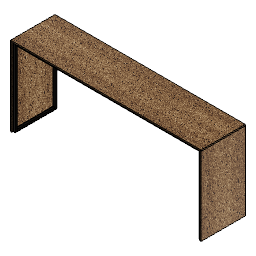
table de lit (Autodesk Fusion 360 design; units mm, degrees)
Autodesk Fusion 360 part; units mm, degrees
sketch "Sketch1" plane through (0, 0, 0) normal (0, 0, 1) x (1, 0, 0) in component "Plateau"
  line L0 (0, 0) -> (1800, 0)
  line L1 (1800, 0) -> (1800, 420)
  line L2 (1800, 420) -> (0, 420)
  line L3 (0, 420) -> (0, 0)
  dimension "d8" = 1800
  dimension "d9" = 420
  constraint horizontal L0
  constraint vertical L1
  constraint horizontal L2
  constraint vertical L3
  constraint coincident L0.start L3.end
  measures "d8" distance of L0.start L0.end
  measures "d9" distance of L0.start L2.end
extrude "Extrude1" add sketch "Sketch1" along normal blind 12 makes body 1 in component "Plateau"
sketch "Sketch1 (2)" plane through (0, 0, 0) normal (0, 0, 1) x (1, 0, 0) in component "Pied"
  line L0 (0, 0) -> (20, 0)
  line L1 (20, 0) -> (20, 20)
  line L2 (20, 20) -> (0, 20)
  line L3 (0, 20) -> (0, 0)
  dimension "d12" = 20
  dimension "d13" = 20
  constraint horizontal L0
  constraint vertical L1
  constraint horizontal L2
  constraint vertical L3
  constraint coincident L0.start L3.end
  measures "d12" distance of L0.start L0.end
  measures "d13" distance of L0.start L2.end
extrude "Extrude1'" add sketch "Sketch1 (2)" along normal blind 738 separate body makes body 2 in component "Pied"
shell "Shell1" thickness 2 removed faces 2 at (6.6667, 13.3333, 738) at (6.6667, 13.3333, 0) on bodies 2 in component "Pied"
pattern_linear "R-Pattern1" count 2 spacing 1756 along (1, 0, 0) count 2 spacing 376 along (0, 1, 0) of bodies 2 makes body 3 at (1756, 13.3333, 246) makes body 4 at (0, 389.3333, 246) makes body 5 at (1756, 389.3333, 246) in component "Pied"
sketch "Sketch2" plane through (0, 0, 738) normal (0, 0, 1) x (-1, 0, 0) in component "Pied"
  line L0 (-2, -18) -> (-18, -18)
  line L1 (-18, -18) -> (-18, -2)
  line L2 (-18, -2) -> (-2, -2)
  line L3 (-2, -2) -> (-2, -18)
  line L4 (0, -20) -> (0, 0)
  line L5 (0, 0) -> (-20, 0)
  line L6 (-20, 0) -> (-20, -20)
  line L7 (-20, -20) -> (0, -20)
  line L8 (-20, -376) -> (-1756, -376) construction
  line L9 (-1756, -376) -> (-1756, -20) construction
  line L10 (-1756, -20) -> (-20, -20) construction
  line L11 (-20, -20) -> (-20, -376) construction
  line L12 (-20, -376) -> (-1756, -20) construction
  line L13 (-1756, -376) -> (-20, -20) construction
  point P0 (-20, -20)
  point P1 (-20, -376)
  point P2 (-1756, -20)
  point P3 (-1756, -376)
  point P4 (-888, -198)
  constraint horizontal L8
  constraint vertical L9
  constraint horizontal L10
  constraint vertical L11
  constraint coincident P2 L9.end
  constraint coincident P1 L8.start
  constraint coincident P3 L8.end
  constraint coincident P0 L6.end
  constraint midpoint L12 P4
sketch "Sketch1 (3)" plane through (0, 0, 0) normal (0, 0, 1) x (1, 0, 0) in component "Plate_side"
  line L0 (0, 0) -> (12, 0)
  line L1 (12, 0) -> (12, 420)
  line L2 (12, 420) -> (0, 420)
  line L3 (0, 420) -> (0, 0)
  dimension "d27" = 12
  dimension "d28" = 420
  constraint horizontal L0
  constraint vertical L1
  constraint horizontal L2
  constraint vertical L3
  constraint coincident L0.start L3.end
  measures "d27" distance of L0.start L0.end
  measures "d28" distance of L0.start L2.end
extrude "Extrude1''" add sketch "Sketch1 (3)" along normal blind 738 separate body makes body 6 in component "Plate_side"
sketch "Sketch2 (2)" plane through (0, 0, 0) normal (0, 0, -1) x (1, 0, 0) in component "Plateau"
  line L0 (0, 0) -> (0, -420)
  line L1 (0, -420) -> (1800, -420)
  line L2 (1800, -420) -> (1800, 0)
  line L3 (1800, 0) -> (0, 0)
  line L4 (0, 0) -> (12, 0) construction
  line L5 (12, 0) -> (12, -420) construction
  line L6 (12, -420) -> (0, -420) construction
  line L7 (0, -420) -> (0, 0) construction
  line L8 (0, -420) -> (12, 0) construction
  line L9 (0, 0) -> (12, -420) construction
  point P0 (6, -210)
  dimension "d31" = 12
  dimension "d32" = 420
  constraint horizontal L4
  constraint vertical L5
  constraint horizontal L6
  constraint vertical L7
  constraint coincident L0.start L3.end
  constraint coincident L0.end L1.start
  constraint midpoint L9 P0
  measures "d31" distance of L0.start L4.end
  measures "d32" distance of L0.start L0.end
pattern_linear "00000000-0000-0000-0000-000000000000" [suppressed]
sketch "Sketch1 (4)" plane through (0, 0, 0) normal (0, 0, -1) x (1, 0, 0)
sketch "Sketch3" plane through (0, 0, 0) normal (0, 0, -1) x (1, 0, 0) in component "Plateau"
  line L0 (1800, 0) -> (1788, 0) construction
  line L1 (1788, 0) -> (1788, -420) construction
  line L2 (1788, -420) -> (1800, -420) construction
  line L3 (1800, -420) -> (1800, 0) construction
  line L4 (1788, -420) -> (1800, 0) construction
  line L5 (1788, 0) -> (1800, -420) construction
  point P0 (1800, 0)
  point P1 (1794, -210)
  dimension "d41" = 12
  dimension "d42" = 420
  constraint horizontal L0
  constraint vertical L1
  constraint horizontal L2
  constraint vertical L3
  constraint coincident P0 L0.start
  constraint midpoint L5 P1
  measures "d41" distance of P0 L0.end
  measures "d42" distance of P0 L2.end
sketch "Sketch4" plane through (32, 0, 0) normal (1, 0, 0) x (0, 1, 0) in component "Plateau"
  line L0 (12, -738) -> (32, -738)
  line L1 (32, -738) -> (32, 0)
  line L2 (32, 0) -> (12, 0)
  line L3 (12, 0) -> (12, -738)
sketch "Sketch1 (5)" plane through (32, 0, 0) normal (1, 0, 0) x (0, 1, 0) in component "main_bar"
  line L0 (12, -738) -> (32, -738)
  line L1 (32, -738) -> (32, 0)
  line L2 (32, 0) -> (12, 0)
  line L3 (12, 0) -> (12, -738)
  line L4 (12, 0) -> (32, 0)
  line L5 (32, 0) -> (32, -20)
  line L6 (32, -20) -> (12, -20)
  line L7 (12, -20) -> (12, 0)
  dimension "d47" = 20
  dimension "d48" = 20
  constraint horizontal L4
  constraint vertical L5
  constraint horizontal L6
  constraint vertical L7
  constraint coincident L2.end L3.start
  measures "d47" distance of L2.end L1.end
  measures "d48" distance of L2.end L6.end
extrude "Extrude1'''" add sketch "Sketch1 (5)" along normal blind 1736 separate body contours L1 L2 L3 L4 L5 L6 L7 makes body 7 in component "main_bar"
shell "Shell1'" thickness 2 removed faces 2 at (1768, 18.6667, -6.6667) at (32, 18.6667, -6.6667) on bodies 7 in component "main_bar"
sketch "Sketch3 (2)" plane through (20, 0, 0) normal (1, 0, 0) x (0, 1, 0) in component "Pied"
  line L0 (0, 0) -> (20, 0)
  line L1 (20, 0) -> (20, 738)
  line L2 (20, 738) -> (0, 738)
  line L3 (0, 738) -> (0, 0)
  line L4 (0, 738) -> (20, 738) construction
  line L5 (20, 738) -> (20, 718) construction
  line L6 (20, 718) -> (0, 718) construction
  line L7 (0, 718) -> (0, 738) construction
  line L8 (0, 738) -> (20, 718) construction
  line L9 (0, 718) -> (20, 738) construction
  point P0 (10, 728)
  dimension "d52" = 20
  dimension "d53" = 20
  constraint horizontal L4
  constraint vertical L5
  constraint horizontal L6
  constraint vertical L7
  constraint coincident L2.end L3.start
  constraint coincident L1.end L2.start
  constraint midpoint L8 P0
  measures "d52" distance of L2.end L1.end
  measures "d53" distance of L2.end L6.end
sketch "Sketch2 (3)" plane through (32, 0, 0) normal (-1, 0, 0) x (0, -1, 0) in component "main_bar"
  line L0 (-14, -2) -> (-14, -18)
  line L1 (-14, -18) -> (-30, -18)
  line L2 (-30, -18) -> (-30, -2)
  line L3 (-30, -2) -> (-14, -2)
  line L4 (-32, -20) -> (-12, -20)
  line L5 (-12, -20) -> (-12, 0)
  line L6 (-12, 0) -> (-32, 0)
  line L7 (-32, 0) -> (-32, -20)
  line L8 (-32, 0) -> (-12, -20) construction
  line L9 (-32, -20) -> (-12, 0) construction
  point P0 (-22, -10)
  constraint coincident L6.end L7.start
  constraint coincident L4.end L5.start
  constraint coincident L4.start L7.end
  constraint coincident L5.end L6.start
  constraint midpoint L9 P0
pattern_linear "00000000-0000-0000-0000-000000000000'" [suppressed]
sketch "Sketch4 (2)" plane through (20, 0, 0) normal (1, 0, 0) x (0, 1, 0) in component "Pied"
  line L0 (376, 0) -> (396, 0)
  line L1 (396, 0) -> (396, 738)
  line L2 (396, 738) -> (376, 738)
  line L3 (376, 738) -> (376, 0)
  line L4 (376, 738) -> (396, 738) construction
  line L5 (396, 738) -> (396, 718) construction
  line L6 (396, 718) -> (376, 718) construction
  line L7 (376, 718) -> (376, 738) construction
  line L8 (376, 738) -> (396, 718) construction
  line L9 (376, 718) -> (396, 738) construction
  point P0 (386, 728)
  dimension "d62" = 20
  dimension "d63" = 20
  constraint horizontal L4
  constraint vertical L5
  constraint horizontal L6
  constraint vertical L7
  constraint coincident L2.end L3.start
  constraint coincident L1.end L2.start
  constraint midpoint L8 P0
  measures "d62" distance of L2.end L1.end
  measures "d63" distance of L2.end L6.end
sketch "Sketch5" plane through (20, 0, 0) normal (1, 0, 0) x (0, 1, 0) in component "Pied"
sketch "Sketch1 (6)" plane through (0, 0, 0) normal (0, 0, 1) x (1, 0, 0) in component "laterral_bar"
  line L0 (0, 0) -> (20, 0)
  line L1 (20, 0) -> (20, 356)
  line L2 (20, 356) -> (0, 356)
  line L3 (0, 356) -> (0, 0)
  dimension "d70" = 20
  dimension "d71" = 356
  constraint horizontal L0
  constraint vertical L1
  constraint horizontal L2
  constraint vertical L3
  constraint coincident L0.start L3.end
  measures "d70" distance of L0.start L0.end
  measures "d71" distance of L0.start L2.end
extrude "Extrude1''''" add sketch "Sketch1 (6)" along normal blind 20 separate body makes body 8 in component "laterral_bar"
shell "Shell1''" thickness 2 removed faces 2 at (13.3333, 356, 6.6667) at (6.6667, 0, 6.6667) on bodies 8 in component "laterral_bar"
sketch "Sketch2 (4)" plane through (0, 356, 0) normal (0, 1, 0) x (-1, 0, 0) in component "laterral_bar"
  line L0 (-2, 18) -> (-2, 2)
  line L1 (-2, 2) -> (-18, 2)
  line L2 (-18, 2) -> (-18, 18)
  line L3 (-18, 18) -> (-2, 18)
  line L4 (-20, 0) -> (0, 0)
  line L5 (0, 0) -> (0, 20)
  line L6 (0, 20) -> (-20, 20)
  line L7 (-20, 20) -> (-20, 0)
  line L8 (-20, 20) -> (0, 0) construction
  line L9 (-20, 0) -> (0, 20) construction
  point P0 (-10, 10)
  constraint coincident L6.end L7.start
  constraint coincident L4.end L5.start
  constraint coincident L4.start L7.end
  constraint coincident L5.end L6.start
  constraint midpoint L9 P0
sketch "Sketch6" plane through (0, 376, 0) normal (0, -1, 0) x (1, 0, 0) in component "Pied"
  line L0 (0, 0) -> (20, 0)
  line L1 (20, 0) -> (20, 738)
  line L2 (20, 738) -> (0, 738)
  line L3 (0, 738) -> (0, 0)
  line L4 (0, 738) -> (20, 738) construction
  line L5 (20, 738) -> (20, 718)
  line L6 (20, 718) -> (0, 718) construction
  line L7 (0, 718) -> (0, 738) construction
  line L8 (0, 738) -> (20, 718) construction
  line L9 (0, 718) -> (20, 738) construction
  point P0 (10, 728)
  dimension "d75" = 20
  dimension "d76" = 20
  constraint horizontal L4
  constraint vertical L5
  constraint horizontal L6
  constraint vertical L7
  constraint coincident L2.end L3.start
  constraint coincident L1.end L2.start
  constraint midpoint L9 P0
  measures "d75" distance of L2.end L1.end
  measures "d76" distance of L2.end L6.end
pattern_linear "00000000-0000-0000-0000-000000000000''" [suppressed] in component "Structure"
component "Coffrage" placed x (1, 0, 0) y (0, 1, 0) z (0, 0, 1) at (0, 0, 0)
component "Structure" placed x (1, 0, 0) y (0, 1, 0) z (0, 0, 1) at (0, 0, 0)
component "Plateau" placed x (1, 0, 0) y (0, 1, 0) z (0, 0, 1) at (0, 0, 0) in component "Coffrage"
component "Plate_side" placed x (1, 0, 0) y (0, 1, 0) z (0, 0, 1) at (0, 0, -738) in component "Coffrage"
component "Plate_side" placed x (1, 0, 0) y (0, 1, 0) z (0, 0, 1) at (1788, 0, -738) in component "Coffrage"
component "Pied" placed x (1, 0, 0) y (0, 1, 0) z (0, 0, 1) at (12, 12, -738) in component "Structure"
component "main_bar" placed x (1, 0, 0) y (0, 1, 0) z (0, 0, 1) at (0, 376, 0) in component "Structure"
component "main_bar" placed x (1, 0, 0) y (0, 1, 0) z (0, 0, 1) at (0, 0, 0) in component "Structure"
component "laterral_bar" placed x (1, 0, 0) y (0, 1, 0) z (0, 0, 1) at (12, 32, -20) in component "Structure"
component "laterral_bar" placed x (1, 0, 0) y (0, 1, 0) z (0, 0, 1) at (12, 32, -738) in component "Structure"
component "laterral_bar" placed x (1, 0, 0) y (0, 1, 0) z (0, 0, 1) at (1768, 32, -20) in component "Structure"
component "laterral_bar" placed x (1, 0, 0) y (0, 1, 0) z (0, 0, 1) at (1768, 32, -738) in component "Structure"
equation "table_length = 1800 mm" comment "Longeur table"
equation "table_width = 420 mm" comment "Largeur table"
equation "table_height = 750 mm" comment "Hauteur table"
equation "table_thickness = 12 mm" comment "Epaisseur de la table"
equation "steel_section = 20 mm" comment "Largeur et profondeur (carree)"
equation "steel_thickness = 2 mm" comment "Epaisseur de l'acier"
equation "d8 = table_length"
equation "d9 = table_width"
equation "d10 = table_thickness"
equation "d12 = steel_section"
equation "d13 = steel_section"
equation "d14 = table_height - table_thickness"
equation "d16 = steel_thickness"
equation "leg_offset = table_thickness" comment "Deport des pieds"
equation "d20 = table_length - 2 * leg_offset - steel_section"
equation "d21 = table_width - 2 * leg_offset - steel_section"
equation "gap_plate = 0 mm" comment "Ecart entre la structure et le plateau"
equation "d27 = table_thickness"
equation "d28 = table_width"
equation "d29 = table_height - table_thickness"
equation "d31 = table_thickness"
equation "d32 = table_width"
equation "d39 = -table_length + table_thickness"
equation "d41 = table_thickness"
equation "d42 = table_width"
equation "d47 = steel_section"
equation "d48 = steel_section"
equation "d49 = table_length - steel_section * 2 - leg_offset * 2"
equation "d51 = steel_thickness"
equation "d52 = steel_section"
equation "d53 = steel_section"
equation "d60 = table_width - steel_section - 2 * leg_offset"
equation "d62 = steel_section"
equation "d63 = steel_section"
equation "d70 = steel_section"
equation "d71 = table_width - 2 * steel_section - 2 * leg_offset"
equation "d72 = steel_section"
equation "d74 = steel_thickness"
equation "d75 = steel_section"
equation "d76 = steel_section"
equation "d83 = -table_height + steel_section + table_thickness"
equation "d84 = table_length - steel_section - 2 * leg_offset"
